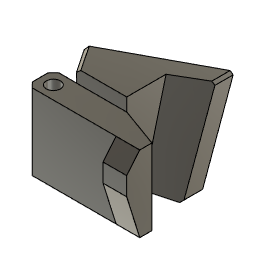
primary_015mm_trigger_L4 (Autodesk Fusion 360 design; units mm, degrees)
Autodesk Fusion 360 part; units mm, degrees
other "Base Mesh Feature1"
sketch "Sketch1" plane through (0, 0, 0) normal (0, 0, 1) x (1, 0, 0)
  circle A0 centre (0, 0) radius 1
  dimension "d1" = 2
  constraint coincident A0.centre origin
  measures "d1" diameter of A0
other "Modify1"
sketch "Sketch2" plane through (0, 0, 0) normal (0, 0, 1) x (1, 0, 0)
  line L0 (10.754932, -10.879876) -> (6.236499, -10.879876)
  line L1 (-9.726628, -3.351367) -> (3.252727, -3.351367)
  line L2 (10.754932, -6.060194) -> (10.754932, -10.879876)
  line L3 (-9.757764, -8.376545) -> (6.236499, -8.376545)
  line L4 (6.236499, -8.376545) -> (6.236499, -10.879876)
  line L5 (-10.747127, -7.381687) -> (-9.757764, -8.376545)
  line L6 (-10.747127, -4.36623) -> (-9.726628, -3.351367)
  line L7 (-10.747127, -7.381687) -> (-10.747127, -4.36623)
  line L8 (3.252727, -3.351367) -> (10.754932, -6.060194)
  line L9 (-8.24857, -2.545864) -> (-8.24857, -9.180715)
  line L10 (-11.529147, -5.865057) -> (-4.824221, -5.865057)
  circle A0 centre (-8.24857, -5.863289) radius 1.339245
  constraint horizontal L0
  constraint horizontal L1
  constraint vertical L2
  constraint horizontal L3
  constraint vertical L4
  constraint perpendicular L5 L6
  constraint perpendicular L3 L9
  constraint perpendicular L9 L10
extrude "Extrude1" add sketch "Sketch2" along normal blind 14.5 contours L0 L1 L2 L3 L4 L8 L9 A0 | L3 L5 L7 L9 L10 A0 | L1 L6 L7 L9 L10 A0 picked at (0.819625, -6.049181) picked at (-9.876624, -7.544727) picked at (-9.86665, -4.18976)
ref_plane "WorkPlane1" through (10.75, 0, 0) normal (1, 0, 0) x (0, 1, 0)
sketch "Sketch3" plane through (10.75, 0, 0) normal (1, 0, 0) x (0, 1, 0)
  line L0 (-8.377256, 14.497171) -> (-11.150034, 14.497171)
  line L1 (-11.150034, 14.497171) -> (-11.150034, 0.000299)
  line L2 (-11.150034, 0.000299) -> (-8.377256, 0.000299)
  line L3 (-8.377256, 0.000299) -> (-8.377256, 14.497171)
  line L4 (-10.868115, 7.995746) -> (-8.377256, 0.000299)
  line L5 (-8.377256, 14.497171) -> (-10.868115, 11.495107)
  line L6 (-10.868115, 11.495107) -> (-10.868115, 7.995746)
  constraint horizontal L0
  constraint vertical L1
  constraint horizontal L2
  constraint vertical L3
  constraint perpendicular L0 L6
extrude "Extrude2" cut sketch "Sketch3" against normal blind 8 contours L0 L1 L2 L4 L5 L6 picked at (-10.131802, 2.665448)
sketch "Sketch4" plane through (0, 0, 14.5) normal (0, 0, 1) x (-1, 0, 0)
  circle A0 centre (8.24857, 5.863289) radius 1.339245
  line L0 (10.747127, 7.381687) -> (9.757764, 8.376545)
  line L1 (9.757764, 8.376545) -> (-6.236499, 8.376545)
  line L2 (-6.236499, 8.376545) -> (-6.236499, 10.879876)
  line L3 (-6.236499, 10.879876) -> (-10.754932, 10.879876)
  line L4 (-10.754932, 10.879876) -> (-10.754932, 6.060194)
  line L5 (-10.754932, 6.060194) -> (-3.252727, 3.351367)
  line L6 (-3.252727, 3.351367) -> (9.726628, 3.351367)
  line L7 (9.726628, 3.351367) -> (10.747127, 4.36623)
  line L8 (10.747127, 4.36623) -> (10.747127, 7.381687)
  line L9 (-10.754932, 10.879876) -> (-6.236499, 10.879876)
  line L10 (-6.236499, 10.879876) -> (-6.236499, 8.376545)
  line L11 (-6.236499, 8.376545) -> (-10.754932, 8.376545)
  line L12 (-10.754932, 8.376545) -> (-10.754932, 10.879876)
  constraint horizontal L9
  constraint vertical L10
  constraint horizontal L11
  constraint vertical L12
extrude "Extrude3" cut sketch "Sketch4" against normal blind 0.01 contours L2 L3 L4 L9 L10 L11 L12 picked at (-7.742643, 10.045432)
extrude "Extrude4" cut 1 faces at (9.2455, -10.045669, 0.000299) along direction (0, 0, -1) blind 1
sketch "Sketch5" plane through (10.754932, 0, 0) normal (1, 0, 0) x (0, 1, 0)
  line L0 (-8.376545, 14.5) -> (-8.376545, 14.49)
  line L1 (-8.376545, 14.49) -> (-10.879876, 14.49)
  line L2 (-10.879876, 14.49) -> (-10.879876, 0)
  line L3 (-10.879876, 0) -> (-6.060194, 0)
  line L4 (-6.060194, 0) -> (-6.060194, 14.5)
  line L5 (-6.060194, 14.5) -> (-8.376545, 14.5)
  line L6 (-8.376545, 14.5) -> (-11.0826, 11.248297)
  line L7 (-11.0826, 11.248297) -> (-11.0826, 14.775026)
  line L8 (-11.0826, 14.775026) -> (-8.416879, 14.775026)
  line L9 (-8.416879, 14.775026) -> (-8.376545, 14.5)
  constraint perpendicular L5 L7
  constraint perpendicular L7 L8
extrude "Extrude5" cut sketch "Sketch5" against normal blind 4.8 contours L1 L2 L6 picked at (-10.048206, 13.490633)
sketch "Sketch6" plane through (10.754932, 0, 0) normal (1, 0, 0) x (0, 1, 0)
  line L0 (-8.384867, 14.49) -> (-10.879876, 11.491898)
  line L1 (-10.879876, 11.491898) -> (-10.879876, 0)
  line L2 (-10.879876, 0) -> (-6.060194, 0)
  line L3 (-6.060194, 0) -> (-6.060194, 14.5)
  line L4 (-6.060194, 14.5) -> (-8.376545, 14.5)
  line L5 (-8.376545, 14.5) -> (-8.376545, 14.49)
  line L6 (-8.376545, 14.49) -> (-8.384867, 14.49)
  line L7 (-8.37122, 0) -> (-10.860947, 8.009289)
  line L8 (-10.860947, 8.009289) -> (-10.983353, 8.009289)
  line L9 (-10.983353, 8.009289) -> (-10.983353, -0.140602)
  line L10 (-10.983353, -0.140602) -> (-8.364126, -0.140602)
  constraint perpendicular L1 L8
  constraint perpendicular L2 L9
  constraint perpendicular L9 L10
extrude "Extrude6" cut sketch "Sketch6" against normal blind 0.01 contours L1 L2 L7 L8 picked at (-10.037348, 2.669763)
sketch "Sketch7" plane through (0, 0, 0) normal (0, 0, 1) x (1, 0, 0)
  line L0 (3.253999, -3.346906) -> (3.253999, -0.239381)
  line L1 (3.253999, -0.239381) -> (9.263309, 1.37584)
  line L2 (9.263309, 1.37584) -> (9.263309, 4.936497)
  line L3 (9.263309, 4.936497) -> (-9.072836, 1.169935)
  line L4 (-9.072836, 1.169935) -> (-6.017309, -3.355961)
  line L5 (-6.017309, -3.355961) -> (3.253999, -3.346906)
  constraint vertical L0
  constraint parallel L0 L2
ref_plane "WorkPlane2" through (0, 0, 17) normal (0, 0, 1) x (1, 0, 0)
sketch "Sketch8" plane through (0, 0, 17) normal (0, 0, 1) x (1, 0, 0)
  line L0 (3.24989, -3.365078) -> (3.24989, 4.15)
  line L1 (3.24989, -3.365078) -> (-6.350298, -3.365078)
  line L2 (-6.350298, -3.365078) -> (-9.350004, 1.135039)
  line L3 (-9.350004, 1.135039) -> (9.249015, 11.142477)
  line L4 (9.249015, 11.142477) -> (9.249015, 7.660005)
  line L5 (9.249015, 7.660005) -> (3.24989, 4.15)
  constraint vertical L0
  constraint perpendicular L0 L1
  constraint perpendicular L1 L4
loft "Loft1" add profiles "Sketch8", "Sketch7" section 1 section 2
chamfer "Chamfer1" distance 0.7 angle 45 1 edges at (-7.850151, -1.11502, 17)
chamfer "Chamfer2" distance 0.4 angle 45 1 edges at (-7.546623, -1.090716, 0)
chamfer "Chamfer3" distance 0.5 angle 45 1 edges at (9.263309, 3.156168, 0)
chamfer "Chamfer4" distance 0.5 angle 45 1 edges at (9.249015, 9.401241, 17)
